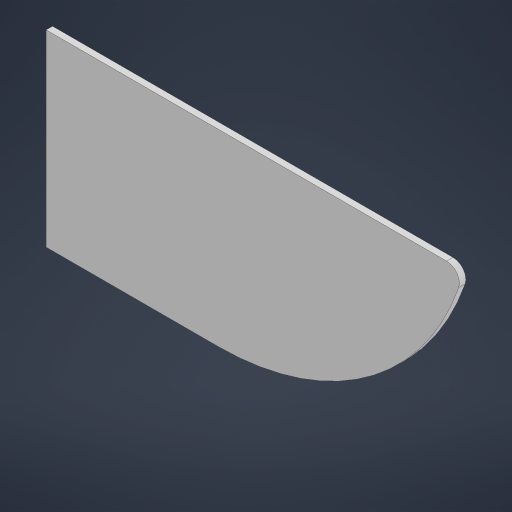
# Autodesk Inventor part: Sleds
Saved by Autodesk Inventor 2023.4 (Build 274418000, 418)
## iProperties
Created: 2023-12-10
Part Number: Sleds
Material: Generic
Document SubType Name: Modeling
Designer: diego
Density: 1 g/cm^3
Appearance: Default
Author: diego
Autodesk Inventor part; units mm, degrees
ref_plane "YZ Plane" through (0, 0, 0) normal (1, 0, 0) x (0, 1, 0)
ref_plane "XZ Plane" through (0, 0, 0) normal (0, 1, 0) x (-1, 0, 0)
ref_plane "XY Plane" through (0, 0, 0) normal (0, 0, 1) x (1, 0, 0)
sketch "Sketch1" plane through (0, 0, 0) normal (0, 0, 1) x (1, 0, 0)
  circle A0 centre (0, 0) radius 63.5
  line L0 (0, 0) -> (63.5, 0)
  line L1 (0, 0) -> (0, -63.5)
  line L2 (0, 0) -> (-127, 0)
  line L3 (-127, 0) -> (-127, -63.5)
  line L4 (-127, -63.5) -> (0, -63.5)
  line L5 (-127, 0) -> (-127, -16.51)
  line L6 (-127, -16.51) -> (61.3161, -16.51)
  dimension "d0" = 127
  dimension "d1" = 127
  dimension "d43" = 16.51
  constraints: 14 end point, 4 perpendicular, 3 point on circle, 1 centre point, 1 coincident, 1 point on line, 1 tangent, 1 vertical
  measures "d0" diameter of A0
  measures "d1" distance of L0.start L2.end
  measures "d43" distance of L2.end L5.end
extrude "Extrusion4" add sketch "Sketch1" along normal blind 1.5875 contours L1 L6 A0 | L4 L3 L6 A0 | A0 L6 L1
sketch "Sketch4" plane through (0, 0, 1.5875) normal (0, 0, 1) x (1, 0, 0)
  arc A0 (0, -63.5) -> (61.3161, -16.51) centre (0, 0) ccw projected
  line L0 (61.3161, -16.51) -> (-59.3339, -16.51)
  line L1 (61.3161, -16.51) -> (-127, -16.51) projected
  line L2 (-59.3339, -16.51) -> (-59.3339, -62.6422)
  line L3 (-59.3339, -62.6422) -> (-59.3339, -63.5)
  line L4 (-127, -63.5) -> (0, -63.5) projected
  line L5 (-136.3806, -11.9346) -> (-59.3339, -11.9346)
  line L6 (-59.3339, -11.9346) -> (-59.3339, -68.0966)
  line L7 (-59.3339, -68.0966) -> (-136.3806, -68.0966)
  line L8 (-136.3806, -68.0966) -> (-136.3806, -11.9346)
  point P0 (-59.3339, -16.51)
  dimension "d46" = 120.65
  constraints: 14 end point, 3 point on line, 2 parallel, 2 perpendicular, 1 horizontal
  measures "d46" distance of L0.start L0.end
extrude "Extrusion5" cut sketch "Sketch4" against normal blind 1.5875 contours L6 L7 L8 L5 L2 L3
fillet "Fillet2" radius 3.175 1 edges at (61.3161, -16.51, 0.7937)
fillet "Fillet3" radius 3.175 2 edges at (-59.3339, -63.5, 0.7937) (-59.3339, -16.51, 0.7937)
sketch "Sketch5" plane through (0, 0, 1.5875) normal (0, 0, 1) x (1, 0, 0)
  circle A0 centre (-55.6881, -20.1151) radius 2.54
  line L0 (-55.6881, -20.1151) -> (-55.6881, -45.5151)
  line L1 (-55.6881, -45.5151) -> (-55.6881, -58.2151)
  circle A1 centre (-55.6881, -58.2151) radius 2.54
  line L2 (-55.6881, -20.1151) -> (-30.2881, -20.1151)
  line L3 (-30.2881, -20.1151) -> (-4.8881, -20.1151)
  line L4 (-4.8881, -20.1151) -> (20.5119, -20.1151)
  line L5 (20.5119, -20.1151) -> (45.9119, -20.1151)
  circle A2 centre (45.9119, -20.1151) radius 2.54
  circle A3 centre (-30.2881, -20.1151) radius 2.54
  circle A4 centre (-4.8881, -20.1151) radius 2.54
  circle A5 centre (20.5119, -20.1151) radius 2.54
  line L6 (-55.6881, -58.2151) -> (-30.2881, -58.2151)
  line L7 (-30.2881, -58.2151) -> (-4.8881, -58.2151)
  line L8 (-4.8881, -58.2151) -> (7.8119, -58.2151)
  circle A6 centre (7.8119, -58.2151) radius 2.54
  circle A7 centre (-30.2881, -58.2151) radius 2.54
  circle A8 centre (-55.6881, -45.5151) radius 2.54
  circle A9 centre (-55.6881, -32.8151) radius 2.54
  line L9 (-59.3339, -12.05) -> (-42.9881, -12.05)
  line L10 (-42.9881, -12.05) -> (-42.9881, -68.751)
  line L11 (-42.9881, -68.751) -> (-59.3339, -68.751)
  line L12 (-59.3339, -68.751) -> (-59.3339, -12.05)
  point P0 (0, 0)
  point P1 (-42.9881, -20.1151)
  point P2 (-42.9881, -58.2151)
  dimension "d51" = 5.08
  dimension "d52" = 25.4
  dimension "d53" = 12.7
  dimension "d54" = 5.08
  dimension "d55" = 25.4
  dimension "d56" = 25.4
  dimension "d57" = 25.4
  dimension "d58" = 25.4
  dimension "d59" = 5.08
  dimension "d60" = 5.08
  dimension "d61" = 5.08
  dimension "d62" = 5.08
  dimension "d63" = 25.4
  dimension "d64" = 25.4
  dimension "d65" = 12.7
  dimension "d66" = 5.08
  dimension "d67" = 5.08
  dimension "d68" = 5.08
  dimension "d69" = 5.08
  constraints: 26 end point, 14 coincident, 10 centre point, 8 horizontal, 3 midpoint, 2 parallel, 2 vertical, 1 perpendicular
  measures "d51" diameter of A0
  measures "d52" distance of L0.start L0.end
  measures "d53" distance of L0.end L1.end
  measures "d54" diameter of A1
  measures "d55" distance of L0.start L2.end
  measures "d56" distance of L3.start L3.end
  measures "d57" distance of L4.start L4.end
  measures "d58" distance of L5.start L5.end
  measures "d59" diameter of A2
  measures "d60" diameter of A3
  measures "d61" diameter of A4
  measures "d62" diameter of A5
  measures "d63" distance of L6.start L6.end
  measures "d64" distance of L7.start L7.end
  measures "d65" distance of L8.start L8.end
  measures "d66" diameter of A6
  measures "d67" diameter of A7
  measures "d68" diameter of A8
  measures "d69" diameter of A9
extrude "Extrusion6" cut sketch "Sketch5" against normal blind 1.5875 contours L2 L0 A0 | L2 L10 L6 A1 L1 A8 L0 A9 A0 | A0 L0 L2 | A0 L0 A9 A8 L1 A1 L6 L10 L11 L12 L9 L2 | A9 L0 | L0 A9 | L6 L1 A1 | A1 L1 L6 | A8 L1 L0 | L0 L1 A8
body "Solid1"
